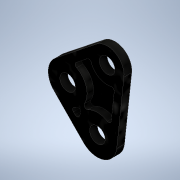
# Autodesk Inventor part: アーム 中間節 先端中詰め
Saved by Autodesk Inventor 2020.2 (Build 242310000, 310)
## iProperties
Created: 2020-05-09
Part Number: アーム 中間節 先端中詰め
Material: ABS プラスチック
Document SubType Name: Modeling
Designer: mozar
Density: 1.06 g/cm^3
Appearance: 滑らか - 黒
Mass: 1.74544 g
Surface Area: 20.239 cm^2
Volume: 1.64664 cm^3
Author: mozar
Autodesk Inventor part; units mm, degrees
ref_plane "YZ Plane" through (0, 0, 0) normal (1, 0, 0) x (0, 1, 0)
ref_plane "XZ Plane" through (0, 0, 0) normal (0, 1, 0) x (-1, 0, 0)
ref_plane "XY Plane" through (0, 0, 0) normal (0, 0, 1) x (1, 0, 0)
sketch "スケッチ1" plane through (0, 0, 0) normal (0, 0, 1) x (1, 0, 0)
  circle A0 centre (-132.6852, 21.2646) radius 3
  circle A1 centre (-105.2485, 37.922) radius 3
  circle A2 centre (-84.1159, 33.5789) radius 3
  circle A3 centre (-77.8119, 54.5794) radius 3
  circle A4 centre (-112.1063, 12.5661) radius 3
  circle A5 centre (-136.4636, -3.8437) radius 3
  circle A6 centre (-147.9517, 7.8722) radius 3
  line L0 (-62.3105, 66.9855) -> (-56.4162, 71.4105)
  line L1 (-56.4162, 71.4105) -> (-60.2332, 71.5281)
  arc A7 (-60.2332, 71.5281) -> (-64.0951, 70.5113) centre (-60.4494, 64.5064) ccw
  line L2 (-64.0951, 70.5113) -> (-153.1544, 16.4415)
  arc A8 (-153.1544, 16.4415) -> (-154.1888, 0.0236) centre (-147.9517, 7.8722) ccw
  line L3 (-154.1888, 0.0236) -> (-141.4408, -10.1069)
  arc A9 (-141.4408, -10.1069) -> (-131.6607, -10.2415) centre (-136.4636, -3.8437) ccw
  line L4 (-131.6607, -10.2415) -> (-40.2316, 58.3956)
  arc A10 (-40.2316, 58.3956) -> (-37.5466, 65.3193) centre (-44.4492, 64.0137) ccw
  line L5 (-37.5466, 65.3193) -> (-62.5812, 46.5254)
  arc A11 (-66.3034, 51.4837) -> (-62.5812, 46.5254) centre (-64.4423, 49.0046) ccw
  line L6 (-66.3034, 51.4837) -> (-41.2688, 70.2776)
  arc A12 (-41.2688, 70.2776) -> (-44.233, 71.0354) centre (-44.4492, 64.0137) ccw
  line L7 (-44.233, 71.0354) -> (-46.496, 71.105)
  line L8 (-46.496, 71.105) -> (-58.5883, 62.0272)
  arc A13 (-62.3105, 66.9855) -> (-58.5883, 62.0272) centre (-60.4494, 64.5064) ccw
  circle A14 centre (-147.9517, 7.8722) radius 1.5
  circle A15 centre (-147.9517, 7.8722) radius 7.5
  circle A16 centre (-136.4636, -3.8437) radius 1.5
  circle A17 centre (-136.4636, -3.8437) radius 7.5
  circle A18 centre (-132.6852, 21.2646) radius 1.5
  circle A19 centre (-132.6852, 21.2646) radius 6.5
  line L9 (-152.6141, 13.7469) -> (-136.7259, 26.3561)
  line L10 (-126.2244, 20.5513) -> (-129.0089, -4.6668)
  line L11 (-153.3068, 2.6212) -> (-141.8187, -9.0947)
  point P0 (0, 0)
  point P1 (0, 0)
  dimension "d0" = 15
  dimension "d1" = 15
  constraints: 24 end point, 20 centre point, 20 point on circle, 7 tangent, 3 coincident
  measures "d0" diameter of A15
  measures "d1" diameter of A17
extrude "押し出し1" add sketch "スケッチ1" against normal blind 3 contours A19 | A19 L10 A17 L11 A15 L9 | A15 | A17
sketch "スケッチ2" plane through (0, 0, 0) normal (0, 0, 1) x (1, 0, 0)
  arc A0 (-152.6141, 13.7469) -> (-153.3068, 2.6212) centre (-147.9517, 7.8722) ccw projected
  line L0 (-153.3068, 2.6212) -> (-141.8187, -9.0947) projected
  arc A1 (-141.8187, -9.0947) -> (-129.0089, -4.6668) centre (-136.4636, -3.8437) ccw projected
  line L1 (-129.0089, -4.6668) -> (-126.2244, 20.5513) projected
  arc A2 (-126.2244, 20.5513) -> (-136.7259, 26.3561) centre (-132.6852, 21.2646) ccw projected
  line L2 (-136.7259, 26.3561) -> (-152.6141, 13.7469) projected
  circle A3 centre (-136.4636, -3.8437) radius 3 projected
  circle A4 centre (-132.6852, 21.2646) radius 3 projected
  circle A5 centre (-147.9517, 7.8722) radius 3 projected
  line L3 (-129.2063, 20.8805) -> (-131.9908, -4.3375)
  arc A6 (-139.6766, -6.9943) -> (-131.9908, -4.3375) centre (-136.4636, -3.8437) ccw
  line L4 (-139.6766, -6.9943) -> (-151.1648, 4.7216)
  arc A7 (-150.7491, 11.397) -> (-151.1648, 4.7216) centre (-147.9517, 7.8722) ccw
  line L5 (-150.7491, 11.397) -> (-134.8609, 24.0062)
  arc A8 (-129.2063, 20.8805) -> (-134.8609, 24.0062) centre (-132.6852, 21.2646) ccw
  arc A9 (-152.6141, 13.7469) -> (-153.3068, 2.6212) centre (-147.9517, 7.8722) ccw projected
  circle A10 centre (-147.9517, 7.8722) radius 7.5
  circle A11 centre (-132.6852, 21.2646) radius 6.5
  circle A12 centre (-136.4636, -3.8437) radius 7.5
  point P0 (0, 0)
  point P1 (-143.8774, -2.7102)
  point P2 (-131.3323, 1.6262)
  point P3 (-129.8074, 15.4364)
  point P4 (-139.1512, 20.6013)
  point P5 (-146.0493, 15.1269)
  point P6 (-146.964, 0.4375)
  dimension "d4" = 3
  constraints: 6 end point, 6 point on circle, 3 centre point, 3 coincident, 14 other
  measures "d4" distance between parallel lines of L1 L3
extrude "押し出し2" cut sketch "スケッチ2" against normal blind 2.5 contours L5 A11 L3 A12 L4 A10
sketch "スケッチ3" plane through (0, 0, 0) normal (0, 0, 1) x (1, 0, 0)
  arc A0 (-146.964, 0.4375) -> (-146.0493, 15.1269) centre (-147.9517, 7.8722) ccw projected
  line L0 (-146.0493, 15.1269) -> (-139.1512, 20.6013) projected
  arc A1 (-139.1512, 20.6013) -> (-129.8074, 15.4364) centre (-132.6852, 21.2646) ccw projected
  line L1 (-129.8074, 15.4364) -> (-131.3323, 1.6262) projected
  arc A2 (-131.3323, 1.6262) -> (-143.8774, -2.7102) centre (-136.4636, -3.8437) ccw projected
  line L2 (-143.8774, -2.7102) -> (-146.964, 0.4375) projected
  arc A3 (-152.6141, 13.7469) -> (-153.3068, 2.6212) centre (-147.9517, 7.8722) ccw projected
  line L3 (-153.3068, 2.6212) -> (-141.8187, -9.0947) projected
  arc A4 (-141.8187, -9.0947) -> (-129.0089, -4.6668) centre (-136.4636, -3.8437) ccw projected
  line L4 (-129.0089, -4.6668) -> (-126.2244, 20.5513) projected
  arc A5 (-126.2244, 20.5513) -> (-136.7259, 26.3561) centre (-132.6852, 21.2646) ccw projected
  line L5 (-136.7259, 26.3561) -> (-152.6141, 13.7469) projected
  circle A6 centre (-136.4636, -3.8437) radius 3 projected
  circle A7 centre (-132.6852, 21.2646) radius 3 projected
  circle A8 centre (-147.9517, 7.8722) radius 3 projected
  arc A9 (-142.9322, -0.048) -> (-144.2837, 1.3303) centre (-143.7947, 0.4581) ccw
  arc A10 (-141.4831, 4.0765) -> (-140.1316, 2.6982) centre (-140.6207, 3.5704) ccw
  point P0 (0, 0)
  dimension "d7" = 2
  dimension "d8" = 2
  constraints: 8 point on circle, 4 tangent, 2 centre point
  measures "d7" diameter of A9
  measures "d8" diameter of A10
extrude "押し出し3" add sketch "スケッチ3" against normal blind 3 contours A0 A10 A2 A9
fillet "フィレット1" radius 1 6 edges at (-146.964, 0.4375, -1.25) (-143.8774, -2.7102, -1.25) (-146.0493, 15.1269, -1.25) (-139.1512, 20.6013, -1.25) (-129.8074, 15.4364, -1.25) (-131.3323, 1.6262, -1.25)
